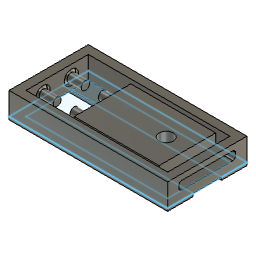
SprVlv v2 (Autodesk Fusion 360 design; units mm, degrees)
Autodesk Fusion 360 part; units mm, degrees
sketch "Sketch1" plane through (0, 0, 0) normal (0, 0, 1) x (1, 0, 0)
  line L0 (0, 0) -> (30, 0)
  line L1 (30, 0) -> (30, 20)
  line L2 (30, 20) -> (0, 20)
  line L3 (0, 20) -> (0, 0)
  circle A0 centre (22.5, 10) radius 2.5
  constraint horizontal L0
  constraint vertical L1
  constraint horizontal L2
  constraint vertical L3
  constraint coincident L0.start L3.end
sketch "Sketch2" plane through (0, 0, 0) normal (1, 0, 0) x (0, 1, 0)
  line L0 (0, 0) -> (20, 0)
  line L1 (20, 0) -> (20, 7)
  line L2 (20, 7) -> (0, 7)
  line L3 (0, 7) -> (0, 0)
  circle A0 centre (15, 3.5) radius 2.5
  circle A1 centre (15, 3.5) radius 1.5
  circle A2 centre (5, 3.5) radius 2.5
  circle A3 centre (5, 3.5) radius 1.5
  constraint horizontal L0
  constraint vertical L1
  constraint horizontal L2
  constraint vertical L3
  constraint coincident L0.start L3.end
  constraint concentric A0 A1
  constraint concentric A2 A3
extrude "Extrude1" add sketch "Sketch1" along normal blind 7 makes body 1
extrude "Extrude2" add sketch "Sketch2" against normal blind 5 contours A1 | A3 bodies 1
extrude "Extrude3" cut sketch "Sketch2" along normal blind 1 contours A0 | A2 bodies 1
sketch "Sketch3" plane through (0, 0, 0) normal (0, 0, 1) x (1, 0, 0)
  line L0 (34, 21) -> (-16, 21)
  line L1 (-16, 21) -> (-16, -1)
  line L2 (-16, -1) -> (34, -1)
  line L3 (34, -1) -> (34, 21)
  line L4 (-19, 24) -> (37, 24)
  line L5 (37, 24) -> (37, -4)
  line L6 (37, -4) -> (-19, -4)
  line L7 (-19, -4) -> (-19, 24)
  constraint horizontal L0
  constraint vertical L1
  constraint horizontal L2
  constraint vertical L3
  constraint horizontal L4
  constraint vertical L5
  constraint horizontal L6
  constraint vertical L7
delete_face "DeleteFace1" 1 faces at (30, 6.6667, 2.3333) on bodies 1
extrude "Extrude5" add sketch "Sketch3" along normal blind 8 separate body makes body 2
move_body "Move1" bodies 1 to x (1, 0, 0) y (0, 1, 0) z (0, 0, 1) at (0, 0, 0.5)
sketch "Sketch5" plane through (0, 0, 0) normal (1, 0, 0) x (0, 1, 0)
  line L0 (20, 7.5) -> (0, 7.5)
  line L1 (0, 7.5) -> (0, 0.5)
  line L2 (0, 0.5) -> (20, 0.5)
  line L3 (20, 0.5) -> (20, 7.5)
  circle A0 centre (15, 4) radius 2.5
  circle A1 centre (15, 4) radius 1.5
  circle A2 centre (5, 4) radius 2.5
  circle A3 centre (5, 4) radius 1.3885
  constraint horizontal L0
  constraint vertical L1
  constraint horizontal L2
  constraint vertical L3
  constraint concentric A0 A1
  constraint concentric A2 A3
extrude "Extrude6" add sketch "Sketch5" along normal blind -16 and the other way blind 11 contours A1 | A3 bodies 2
extrude "Extrude7" cut sketch "Sketch5" against normal blind 17 contours A0 | A2 bodies 2
sketch "Sketch6" plane through (0, 0, 0) normal (1, 0, 0) x (0, 1, 0)
  line L0 (0, 6) -> (20, 6)
  line L1 (20, 6) -> (20, 3)
  line L2 (20, 3) -> (0, 3)
  line L3 (0, 3) -> (0, 6)
  constraint horizontal L0
  constraint vertical L1
  constraint horizontal L2
  constraint vertical L3
extrude "Extrude8" cut sketch "Sketch6" along normal blind 43 bodies 2
sketch "Sketch7" plane through (0, 0, 0) normal (0, 0, 1) x (1, 0, 0)
  line L0 (-19, -4) -> (37, -4)
  line L1 (37, -4) -> (37, 5)
  line L2 (37, 5) -> (-19, 5)
  line L3 (-19, 5) -> (-19, -4)
  line L4 (37, 24) -> (-19, 24)
  line L5 (-19, 24) -> (-19, 15)
  line L6 (-19, 15) -> (37, 15)
  line L7 (37, 15) -> (37, 24)
  constraint horizontal L0
  constraint vertical L1
  constraint horizontal L2
  constraint vertical L3
  constraint horizontal L4
  constraint vertical L5
  constraint horizontal L6
  constraint vertical L7
extrude "Extrude9" add sketch "Sketch7" against normal blind 1 bodies 2
fillet "Fillet1" radius 1 2 edges at (35.5, 20, 6) (35.5, 20, 3) on bodies 2
fillet "Fillet2" radius 1 2 edges at (35.5, 0, 6) (35.5, 0, 3) on bodies 2
fillet "Fillet3" radius 1 2 edges at (-17, 3.7054, 3.4979) (-17, 13.6015, 3.4576) on bodies 2
fillet "Fillet4" radius 1 2 edges at (1, 13.6015, 4.5424) (1, 3.6015, 4.5424) on bodies 1
